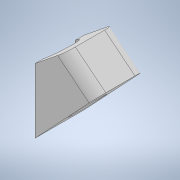
# Autodesk Inventor part: My really cool, really epic hole in a ramp
Saved by Autodesk Inventor 2022 (Build 260153000, 153)
## iProperties
Created: 2022-10-06
Part Number: My really cool, really epic hole in a ramp
Material: Generic
Document SubType Name: Modeling
Designer: c2067183
Density: 1 g/cm^3
Appearance: Default
Author: c2067183
Autodesk Inventor part; units mm, degrees
ref_plane "YZ Plane" through (0, 0, 0) normal (1, 0, 0) x (0, 1, 0)
ref_plane "XZ Plane" through (0, 0, 0) normal (0, 1, 0) x (-1, 0, 0)
ref_plane "XY Plane" through (0, 0, 0) normal (0, 0, 1) x (1, 0, 0)
sketch "Sketch1" plane through (0, 0, 0) normal (0, 0, 1) x (1, 0, 0)
  line L0 (0, 0) -> (6.1915, 5.0087)
  line L1 (6.1915, 5.0087) -> (12.383, 0)
  line L2 (12.383, 0) -> (0, -13.1985)
  line L3 (0, -13.1985) -> (0, 0)
  point P0 (5.6638, -7.1617)
  dimension "d2" = 7.854
  dimension "d3" = 7.9638
  dimension "d4" = 18.0981
  constraints: 8 end point, 1 vertical
  measures "d2" angle of L2 L0
  measures "d3" distance of L0.start L0.end
  measures "d4" distance of L1.end L2.end
extrude "Extrusion1" add sketch "Sketch1" along normal blind 10
sketch "Sketch3" plane through (0, 0, 10) normal (-0.6289, 0.7775, 0) x (0, 0, -1)
  circle A0 centre (4.9487, 0) radius 3.2373
  point P0 (10, 0)
  constraints: 1 centre point, 1 horizontal alignment
extrude "Extrusion2" cut sketch "Sketch3" against normal blind 10
fillet "Fillet1" radius 2.02 2 edges at (9.2873, 2.5044, 10) (9.2873, 2.5044, 0)
body "Solid1"
